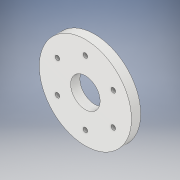
# Autodesk Inventor part: SJ006
Saved by Autodesk Inventor 2017 SP1 (Build 210196100, 196)
## iProperties
Created: 2017-06-04
Part Number: SJ006
Material: ABS Plastic
Document SubType Name: Modeling
Designer: Zach
Density: 1.06 g/cm^3
Appearance: CR White
Author: Zach
Autodesk Inventor part; units mm, degrees
ref_plane "YZ Plane" through (0, 0, 0) normal (1, 0, 0) x (0, 1, 0)
ref_plane "XZ Plane" through (0, 0, 0) normal (0, 1, 0) x (-1, 0, 0)
ref_plane "XY Plane" through (0, 0, 0) normal (0, 0, 1) x (1, 0, 0)
sketch "Sketch1" plane through (0, 0, 0) normal (0, 0, 1) x (1, 0, 0)
  circle A0 centre (0, 0) radius 50
  circle A1 centre (0, 0) radius 16
  dimension "d0" = 100
  dimension "d1" = 32
  constraints: 2 centre point, 2 coincident
  measures "d0" diameter of A0
  measures "d1" diameter of A1
extrude "Extrusion1" add sketch "Sketch1" along normal blind 10
sketch "Sketch2" plane through (0, 0, 10) normal (0, 0, 1) x (1, 0, 0)
  circle A0 centre (0, 35) radius 2.5
  circle A1 centre (-30.3109, 17.5) radius 2.5
  circle A2 centre (-30.3109, -17.5) radius 2.5
  circle A3 centre (0, -35) radius 2.5
  circle A4 centre (30.3109, -17.5) radius 2.5
  circle A5 centre (30.3109, 17.5) radius 2.5
  point P0 (0, 0)
  dimension "d4" = 5
  dimension "d5" = 35
  dimension "d8" = 360
  constraints: 6 centre point, 1 vertical alignment, 13 other
  measures "d4" diameter of A0
  measures "d5" distance of point (0, 0) A0.centre
extrude "Extrusion2" cut sketch "Sketch2" against normal through all
body "Solid1"
